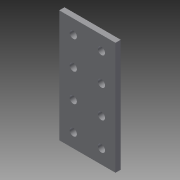
# Autodesk Inventor part: 4165
Saved by Autodesk Inventor 2014 SP2 (Build 180246200, 246)
## iProperties
Created: 2019-11-07
Part Number: 4165
Material: Generic
Catalog Web Link: www.cadenas.de
Description: 4165, 4365, 4165-Black, 4365-Black-Joining Plates - 8 Hole Joining Plate
Vendor: 8020
Document SubType Name: Modeling
Designer: psadmin
Manufacturer: 8020
Mass: 23.3676 g
Surface Area: 120.26 cm^2
Volume: 23.3676 cm^3
Density: 1 g/cm^3
Appearance: PSOLRGB-191-191-191
Category: PARTsolutions
Company: 8020
Title: 4165
Author: Cadenas PARTsolutions
Comments: Joining Plates - 8 Hole Joining Plate
PSOL_IDENT_0: {$CADENAS_DATA\23d-libs\8020\inch\joining_plates\4165.prj},176 {VTYP=3D},{NB=4165},{LINA=4165},{NN=4
PSOL_IDENT_1: 165, 4365, 4165-Black, 4365-Black},{DATE=01.10.2019 06:04:23},{GEOMDATE=11.07.2017 14:50:59},{VERSIO
PSOL_IDENT_2: N=},{LINEID=10},{WBVAR=},{WBNUMERIC=}  {NB=4165},{LINA=4165},{KT=DUMMY},{PN=4165},{A=2.000},{B=4.000
PSOL_IDENT_3: },{F=0.257},{W=.140},{A1=0.5000},{C1=1.500},{C2=0.500},{C3=2.500},{C4=3.500},{D1=0.188},{COLOR=.75,.
PSOL_IDENT_4: 75,.75}
NN: 4165, 4365, 4165-Black, 4365-Black
NT: Joining Plates - 8 Hole Joining Plate
NB: 4165
NBSYN: $PN.
LINA: 4165
PN: 4165
A: 2
B: 4
W: .140
SUPPLIER: 8020
ARTICLENO: 4165
BOMINFO: 4165
CREATOR: CADENAS GmbH
Autodesk Inventor part; units mm, degrees
ref_plane "YZ Plane" through (0, 0, 0) normal (1, 0, 0) x (0, 1, 0)
ref_plane "XZ Plane" through (0, 0, 0) normal (0, 1, 0) x (-1, 0, 0)
ref_plane "XY Plane" through (0, 0, 0) normal (0, 0, 1) x (1, 0, 0)
sketch "Sketch_1" plane through (0, 0, 0) normal (0, 0, 1) x (1, 0, 0)
  line L0 (-25.4, 101.6) -> (-25.4, 0)
  line L1 (-25.4, 0) -> (25.4, 0)
  line L2 (25.4, 0) -> (25.4, 101.6)
  line L3 (25.4, 101.6) -> (-25.4, 101.6)
  circle A0 centre (12.7, 12.7) radius 3.2639
  circle A1 centre (12.7, 38.1) radius 3.2639
  circle A2 centre (12.7, 63.5) radius 3.2639
  circle A3 centre (12.7, 88.9) radius 3.2639
  circle A4 centre (-12.7, 12.7) radius 3.2639
  circle A5 centre (-12.7, 38.1) radius 3.2639
  circle A6 centre (-12.7, 63.5) radius 3.2639
  circle A7 centre (-12.7, 88.9) radius 3.2639
  constraints: 8 centre point, 8 end point
extrude "Extrusion1" add sketch "Sketch_1" along normal blind 4.7752
body "Solid1"
